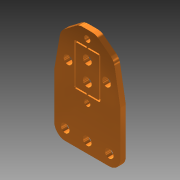
# Autodesk Inventor part: Standard Sensor Mount
Saved by Autodesk Inventor 2022 (Build 260153000, 153)
## iProperties
Created: 2022-02-13
Part Number: Standard Sensor Mount
Material: Aluminum 6061
Document SubType Name: Sheet Metal
Designer: Desktop
Density: 2.7 g/cm^3
Appearance: Metal 1600F Hot
Sheet Metal Rule: Default
Author: Desktop
Autodesk Inventor part; units mm, degrees
ref_plane "YZ Plane" through (0, 0, 0) normal (1, 0, 0) x (0, 1, 0)
ref_plane "XZ Plane" through (0, 0, 0) normal (0, 1, 0) x (-1, 0, 0)
ref_plane "XY Plane" through (0, 0, 0) normal (0, 0, 1) x (1, 0, 0)
sketch "Sketch1" plane through (0, 0, 0) normal (0, 0, 1) x (1, 0, 0)
  line L0 (19.05, 12.7) -> (-19.05, 12.7)
  line L1 (-19.05, 12.7) -> (-19.05, -12.7)
  line L2 (-19.05, -12.7) -> (19.05, -12.7)
  line L3 (19.05, -12.7) -> (19.05, 12.7)
  circle A0 centre (-12.7, 0) radius 2.4892
  line L4 (-12.7, 0) -> (12.7, 0)
  circle A1 centre (12.7, 0) radius 2.4892
  line L5 (-19.05, -6.35) -> (19.05, -6.35)
  circle A2 centre (-11.1125, 34.925) radius 2.4892
  line L6 (-11.1125, 34.925) -> (11.1125, 34.925)
  circle A3 centre (11.1125, 34.925) radius 2.4892
  line L7 (-19.05, 12.7) -> (-19.05, 26.343)
  line L8 (-19.05, 26.343) -> (-15.3495, 47.625)
  line L9 (-15.3495, 47.625) -> (15.3495, 47.625)
  line L10 (15.3495, 47.625) -> (19.05, 26.343)
  line L11 (19.05, 26.343) -> (19.05, 12.7)
  circle A4 centre (-11.1125, 34.925) radius 6.35 construction
  circle A5 centre (0, 29.425) radius 2.54
  circle A6 centre (0, 40.425) radius 2.54
  line L12 (0, 40.425) -> (0, 29.425)
  circle A7 centre (0, 0) radius 2.4892
  line L13 (7.493, 46.99) -> (-7.493, 46.99)
  line L14 (-7.493, 46.99) -> (-7.493, 22.86)
  line L15 (-7.493, 22.86) -> (7.493, 22.86)
  line L16 (7.493, 22.86) -> (7.493, 46.99)
  line L17 (7.493, 46.99) -> (-7.493, 22.86) construction
  line L18 (-7.493, 46.99) -> (7.493, 22.86) construction
  circle A8 centre (0, 50.925) radius 1.778
  circle A9 centre (0, 18.925) radius 1.778
  line L19 (-15.3495, 47.625) -> (-4.7625, 55.6875)
  line L20 (4.7625, 55.6875) -> (15.3495, 47.625)
  line L21 (-7.493, 34.925) -> (7.493, 34.925) construction
  line L22 (-7.493, 37.3062) -> (7.493, 37.3062)
  line L23 (-7.493, 34.1313) -> (7.493, 34.1313)
  line L24 (4.7625, 55.6875) -> (-4.7625, 55.6875)
  line L25 (7.493, 37.3062) -> (7.493, 34.1313)
  line L26 (-7.493, 37.3062) -> (-7.493, 34.1313)
  line L27 (-6.6992, 46.1963) -> (6.6992, 46.1963)
  line L28 (6.6992, 46.1963) -> (6.6992, 23.6537)
  line L29 (6.6992, 23.6537) -> (-6.6992, 23.6537)
  line L30 (-6.6992, 23.6537) -> (-6.6992, 46.1963)
  line L31 (0.254, 46.99) -> (-0.254, 46.99)
  line L32 (-0.254, 46.99) -> (-0.254, 46.1963)
  line L33 (-0.254, 46.1963) -> (0.254, 46.1963)
  line L34 (0.254, 46.1963) -> (0.254, 46.99)
  line L35 (0.254, 46.99) -> (-0.254, 46.1963) construction
  line L36 (-0.254, 46.99) -> (0.254, 46.1963) construction
  line L37 (0.254, 22.86) -> (-0.254, 22.86)
  line L38 (-0.254, 22.86) -> (-0.254, 23.6537)
  line L39 (-0.254, 23.6537) -> (0.254, 23.6537)
  line L40 (0.254, 23.6537) -> (0.254, 22.86)
  line L41 (0.254, 22.86) -> (-0.254, 23.6537) construction
  line L42 (-0.254, 22.86) -> (0.254, 23.6537) construction
  point P0 (0, 12.7)
  point P1 (0, 47.625)
  point P2 (0, 34.925)
  point P3 (0, 34.925)
  point P4 (0, 34.925)
  point P5 (-7.493, 34.1313)
  point P6 (7.493, 34.1313)
  point P7 (7.493, 37.3062)
  point P8 (-7.493, 37.3062)
  point P9 (0, 55.6875)
  point P10 (0, -12.7)
  point P11 (0, 46.5931)
  point P12 (0, 46.5931)
  point P13 (0, 23.2569)
  point P14 (0, 23.2569)
  dimension "d0" = 38.1
  dimension "d1" = 25.4
  dimension "d2" = 4.9784
  dimension "d3" = 4.9784
  dimension "d4" = 25.4
  dimension "d5" = 6.35
  dimension "d6" = 4.9784
  dimension "d7" = 22.225
  dimension "d8" = 22.225
  dimension "d9" = 21.282
  dimension "d10" = 12.7
  dimension "d11" = 12.7
  dimension "d12" = 5.08
  dimension "d13" = 11
  dimension "d17" = 24.13
  dimension "d18" = 14.986
  dimension "d19" = 3.556
  dimension "d22" = 360
  dimension "d24" = 32
  dimension "d29" = 0.7937
  dimension "d31" = 3.175
  dimension "d32" = 4.7625
  dimension "d33" = 9.525
  dimension "d51" = 12.7
  dimension "d52" = 6.35
  dimension "d53" = 0.7937
  dimension "d54" = 0.508
  constraints: 88 end point, 18 midpoint, 11 parallel, 10 centre point, 6 horizontal, 6 perpendicular, 6 symmetric about line, 6 vertical alignment, 5 point on line, 4 coincident, 3 equal length, 3 equal radius, 2 collinear, 1 tangent, 1 vertical, 8 other
  measures "d0" distance of L2.end L1.end
  measures "d1" distance of L1.end L0.end
  measures "d2" diameter of A0
  measures "d3" diameter of A1
  measures "d4" distance of L4.start L4.end
  measures "d5" distance between parallel lines of L2 L5
  measures "d6" diameter of A2
  measures "d7" distance of L6.start L6.end
  measures "d8" distance between parallel lines of L0 L6
  measures "d9" distance from line of L10.end L9
  measures "d10" diameter of A4
  measures "d11" distance from line of L6.start L9
  measures "d12" diameter of A6
  measures "d13" distance of L12.start L12.end
  measures "d17" distance of L14.end L13.end
  measures "d18" distance between parallel lines of L16 L14
  measures "d19" diameter of A8
  measures "d24" distance of A8.centre A9.centre
  measures "d29" distance between parallel lines of L6 L23
  measures "d31" distance between parallel lines of L23 L22
  measures "d32" distance from line of A8.centre L24
  measures "d33" distance of L20.start L19.end
  measures "d51" distance from line of L4.start L0
  measures "d52" distance from line of L4.start L5
  measures "d53" distance between parallel lines of L13 L27
  measures "d54" distance between parallel lines of L32 L34
extrude "Plate1" add sketch "Sketch1" along normal blind 3.175 contours L3 L5 L1 L0 | L0 L7 L8 L9 L10 L11 | L9 L19 L24 L20 | L30 L22 L12 L6 | L6 L12 L23 L30 | L12 L22 L28 L6 | L6 L28 L23 L12 | L23 L28 L29 L30 | L30 L27 L28 L22 | L13 L34 L27 L32 | L38 L29 L40 L15
fillet "Corner Round2" radius 6.35 8 edges at (19.05, -6.35, 1.5875) (-19.05, -6.35, 1.5875) (19.05, 26.343, 1.5875) (-15.3495, 47.625, 1.5875) (-4.7625, 55.6875, 1.5875) (4.7625, 55.6875, 1.5875) (15.3495, 47.625, 1.5875) (-19.05, 26.343, 1.5875)
cut "Cut1" [suppressed]
fillet "Corner Round3" radius 0.7937 4 edges at (-7.493, 46.99, 1.5875) (-7.493, 22.86, 1.5875) (7.493, 22.86, 1.5875) (7.493, 46.99, 1.5875)
fillet "Corner Round4" radius 0.3969 4 edges at (6.6992, 46.1963, 1.5875) (-6.6992, 46.1963, 1.5875) (-6.6992, 23.6537, 1.5875) (6.6992, 23.6537, 1.5875)
sketch "Sketch4" plane through (0, 0, 3.175) normal (0, 0, 1) x (1, 0, 0)
  line L0 (0.254, 46.99) -> (6.6992, 46.99) projected
  arc A0 (7.493, 46.1963) -> (6.6992, 46.99) centre (6.6992, 46.1963) ccw projected
  line L1 (7.493, 46.1963) -> (7.493, 23.6538) projected
  arc A1 (6.6992, 22.86) -> (7.493, 23.6538) centre (6.6992, 23.6538) ccw projected
  line L2 (6.6992, 22.86) -> (0.254, 22.86) projected
  arc A2 (-7.493, 23.6538) -> (-6.6993, 22.86) centre (-6.6993, 23.6538) ccw projected
  line L3 (-7.493, 23.6538) -> (-7.493, 46.1963) projected
  arc A3 (-6.6993, 46.99) -> (-7.493, 46.1963) centre (-6.6993, 46.1963) ccw projected
  arc A4 (-18.9561, 26.8828) -> (-19.05, 25.795) centre (-12.7, 25.795) ccw projected
  line L4 (-19.05, 0) -> (-19.05, 25.795) projected
  arc A5 (-19.05, 0) -> (-12.7, -6.35) centre (-12.7, 0) ccw projected
  line L5 (12.7, -6.35) -> (-12.7, -6.35) projected
  arc A6 (12.7, -6.35) -> (19.05, 0) centre (12.7, 0) ccw projected
  line L6 (19.05, 25.795) -> (19.05, 0) projected
  arc A7 (19.05, 25.795) -> (18.9561, 26.8828) centre (12.7, 25.795) ccw projected
  line L7 (15.7763, 45.1704) -> (18.9561, 26.8828) projected
  arc A8 (15.7763, 45.1704) -> (13.3674, 49.1345) centre (9.5202, 44.0826) ccw projected
  line L8 (6.4671, 54.3894) -> (13.3674, 49.1345) projected
  arc A9 (6.4671, 54.3894) -> (2.6199, 55.6875) centre (2.6199, 49.3375) ccw projected
  line L9 (-2.6199, 55.6875) -> (2.6199, 55.6875) projected
  arc A10 (-2.6199, 55.6875) -> (-6.4671, 54.3894) centre (-2.6199, 49.3375) ccw projected
  line L10 (-13.3674, 49.1345) -> (-6.4671, 54.3894) projected
  arc A11 (-13.3674, 49.1345) -> (-15.7763, 45.1704) centre (-9.5202, 44.0826) ccw projected
  line L11 (-18.9561, 26.8828) -> (-15.7763, 45.1704) projected
  circle A12 centre (11.1125, 34.925) radius 2.4892 projected
  circle A13 centre (-11.1125, 34.925) radius 2.4892 projected
  circle A14 centre (0, 18.925) radius 1.778 projected
  circle A15 centre (0, 0) radius 2.4892 projected
  circle A16 centre (12.7, 0) radius 2.4892 projected
  circle A17 centre (-12.7, 0) radius 2.4892 projected
  circle A18 centre (0, 50.925) radius 1.778 projected
  line L12 (-27.7407, 9.4742) -> (24.6669, 9.4742)
  arc A19 (-11.4438, 46.6085) -> (-12.6483, 44.6265) centre (-9.5202, 44.0826) ccw
  line L13 (-11.4438, 46.6085) -> (-4.5435, 51.8634)
  arc A20 (-2.6199, 52.5125) -> (-4.5435, 51.8634) centre (-2.6199, 49.3375) ccw
  line L14 (-2.6199, 52.5125) -> (2.6199, 52.5125)
  arc A21 (4.5435, 51.8634) -> (2.6199, 52.5125) centre (2.6199, 49.3375) ccw
  line L15 (4.5435, 51.8634) -> (11.4438, 46.6085)
  arc A22 (12.6483, 44.6265) -> (11.4438, 46.6085) centre (9.5202, 44.0826) ccw
  line L16 (12.6483, 44.6265) -> (15.8281, 26.3389)
  arc A23 (15.875, 25.795) -> (15.8281, 26.3389) centre (12.7, 25.795) ccw
  line L17 (15.875, 25.795) -> (15.875, 0)
  arc A24 (12.7, -3.175) -> (15.875, 0) centre (12.7, 0) ccw
  line L18 (12.7, -3.175) -> (-12.7, -3.175)
  arc A25 (-15.875, 0) -> (-12.7, -3.175) centre (-12.7, 0) ccw
  line L19 (-15.875, 0) -> (-15.875, 25.795)
  arc A26 (-15.8281, 26.3389) -> (-15.875, 25.795) centre (-12.7, 25.795) ccw
  line L20 (-15.8281, 26.3389) -> (-12.6483, 44.6265)
  line L21 (-8.6233, 15.877) -> (8.6233, 15.877)
  line L22 (8.6233, 15.877) -> (15.8281, 26.3389)
  line L23 (-8.6233, 15.877) -> (-15.8281, 26.3389)
  line L24 (-8.6233, 15.877) -> (-8.6233, 5.6134)
  line L25 (-8.6233, 5.6134) -> (-15.875, 5.6134)
  line L26 (8.6233, 15.877) -> (8.6233, 5.6134)
  line L27 (8.6233, 5.6134) -> (15.875, 5.6134)
  line L28 (-10.0711, 17.9793) -> (-10.0711, 5.6134)
  line L29 (10.0711, 17.9793) -> (10.0711, 5.6134)
  arc A27 (6.3024, 23.6537) -> (6.6992, 24.0506) centre (6.3024, 24.0506) ccw projected
  line L30 (6.6992, 45.7994) -> (6.6992, 24.0506) projected
  arc A28 (6.6992, 45.7994) -> (6.3024, 46.1963) centre (6.3024, 45.7994) ccw projected
  line L31 (0.254, 46.1963) -> (6.3024, 46.1963) projected
  line L32 (0.254, 46.99) -> (0.254, 46.1963) projected
  line L33 (0.254, 23.6537) -> (0.254, 22.86) projected
  line L34 (6.3024, 23.6537) -> (0.254, 23.6537) projected
  arc A29 (-6.6992, 24.0506) -> (-6.3024, 23.6537) centre (-6.3024, 24.0506) ccw projected
  line L35 (-0.254, 23.6537) -> (-6.3024, 23.6537) projected
  line L36 (-0.254, 22.86) -> (-0.254, 23.6537) projected
  line L37 (-0.254, 22.86) -> (-6.6993, 22.86) projected
  line L38 (-6.6993, 46.99) -> (-0.254, 46.99) projected
  line L39 (-0.254, 46.1963) -> (-0.254, 46.99) projected
  line L40 (-6.3024, 46.1963) -> (-0.254, 46.1963) projected
  arc A30 (-6.3024, 46.1963) -> (-6.6992, 45.7994) centre (-6.3024, 45.7994) ccw projected
  line L41 (-6.6992, 24.0506) -> (-6.6992, 45.7994) projected
  point P0 (0, 15.877)
  dimension "d59" = 9.4742
  dimension "d60" = 3.175
  dimension "d61" = 17.2466
  dimension "d62" = 3.048
  dimension "d63" = 1.4478
  dimension "d67" = 5.6134
  constraints: 36 end point, 16 point on circle, 8 centre point, 7 point on line, 3 perpendicular, 2 horizontal, 2 vertical, 1 collinear, 1 midpoint, 1 parallel, 1 vertical alignment, 15 other
  measures "d59" distance from line of point (0, 0) L12
  measures "d60" distance between parallel lines of L11 L20
  measures "d61" distance of L21.start L21.end
  measures "d62" distance from line of A14.centre L21
  measures "d63" distance between parallel lines of L26 L29
  measures "d67" distance from line of A6.centre L27
cut "Cut2" [suppressed]
feature "Corner Round5" [suppressed]
equation "\"d55\" = Thickness"
equation "\"d64\" = Thickness"
equation "\"d35\" = Thickness"
equation "\"BendReliefWidth\" = Thickness"
equation "\"BendReliefDepth\" = 0.5 * Thickness"
equation "\"CornerReliefSize\" = 4 * Thickness"
equation "\"MinimumRemnant\" = 2 * Thickness"
equation "\"TransitionRadius\" = BendRadius"
equation "\"JacobiRadiusSize\" = BendRadius"
equation "\"GapSize\" = Thickness"
equation "\"Thickness\" = 3.175"
equation "\"BendRadius\" = 0.79375"
body "Solid1"
